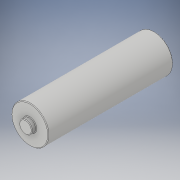
# Autodesk Inventor part: battery
Saved by Autodesk Inventor 2019 (Build 230136000, 136)
## iProperties
Created: 2020-11-03
Part Number: battery
Material: 一般
Document SubType Name: Modeling
Designer: masato
Density: 1 g/cm^3
Appearance: 既定
Author: masato
## iProperties of the stored document battery_3D プリント.ipt
Created: 2020-11-03
Part Number: battery_3D プリント
Material: 一般
Document SubType Name: Modeling
Designer: masato
Density: 1 g/cm^3
Appearance: 既定
Author: masato
Autodesk Inventor part; units mm, degrees
ref_plane "YZ Plane" through (0, 0, 0) normal (1, 0, 0) x (0, 1, 0)
ref_plane "XZ Plane" through (0, 0, 0) normal (0, 1, 0) x (-1, 0, 0)
ref_plane "XY Plane" through (0, 0, 0) normal (0, 0, 1) x (1, 0, 0)
sketch "スケッチ1" plane through (0, 0, 0) normal (0, 0, 1) x (1, 0, 0)
  circle A0 centre (0, 0) radius 7.25
  dimension "d0" = 14.5
  constraints: 1 centre point, 1 coincident
  measures "d0" diameter of A0
extrude "押し出し1" add sketch "スケッチ1" along normal blind 48.8
sketch "スケッチ2" plane through (0, 0, 48.8) normal (0, 0, 1) x (1, 0, 0)
  circle A0 centre (0, 0) radius 2.5
  dimension "d3" = 5
  constraints: 1 centre point, 1 coincident
  measures "d3" diameter of A0
extrude "押し出し2" add sketch "スケッチ2" along normal blind 1.7
fillet "フィレット1" radius 0.25 4 edges at (-7.25, 0, 48.8) (-7.25, 0, 0) (-2.5, 0, 50.5) (-2.5, 0, 48.8)
